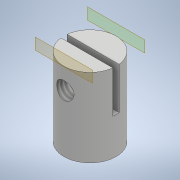
# Autodesk Inventor part: slit-adapter-clear-scope_8_2018
Saved by Autodesk Inventor 2021 (Build 250183000, 183)
## iProperties
Created: 2018-04-16
Part Number: slit-adapter-clear-scope_8_2018
Material: Generic
Document SubType Name: Modeling
Designer: FiolkaLab
Density: 1 g/cm^3
Appearance: Default
Author: FiolkaLab
Autodesk Inventor part; units mm, degrees
ref_plane "YZ Plane" through (0, 0, 0) normal (1, 0, 0) x (0, 1, 0)
ref_plane "XZ Plane" through (0, 0, 0) normal (0, 1, 0) x (-1, 0, 0)
ref_plane "XY Plane" through (0, 0, 0) normal (0, 0, 1) x (1, 0, 0)
sketch "Sketch1" plane through (0, 0, 0) normal (0, 0, 1) x (1, 0, 0)
  circle A0 centre (0, 0) radius 5
  dimension "d0" = 10
  constraints: 1 centre point, 1 coincident
  measures "d0" diameter of A0
extrude "Extrusion1" add sketch "Sketch1" along normal blind 15
sketch "Sketch2" plane through (0, 0, 15) normal (0, 0, 1) x (1, 0, 0)
  line L0 (-4.9749, -0.5) -> (4.9749, -0.5)
  line L1 (4.9749, -0.5) -> (4.9749, 0.5)
  line L2 (4.9749, 0.5) -> (-4.9749, 0.5)
  line L3 (-4.9749, 0.5) -> (-4.9749, -0.5)
  circle A0 centre (0, 0) radius 5 projected
  dimension "d3" = 1
  constraints: 8 end point, 3 point on circle, 2 parallel, 1 horizontal, 1 perpendicular
  measures "d3" distance of L2.end L0.start
sketch "Sketch3" plane through (0, 0, 0) normal (0, 0, -1) x (-1, 0, 0)
  circle A0 centre (0, 0) radius 1.4142
  constraints: 1 centre point, 1 coincident
hole "Hole1" at (0, 0, 0) direction (0, 0, 1) diameter 3.302 depth 7 thread size "8-32 UNC" class "2B" standard "ANSI Unified Screw Threads"
extrude "Extrusion2" add sketch "Sketch2" along normal blind 2 contours L3 L2 L1 L0
ref_plane "Work Plane1" through (-4.9749, 5, 15) normal (0, 1, 0) x (1, 0, 0)
ref_plane "Work Plane2" through (-4.9749, -5, 15) normal (0, -1, 0) x (1, 0, 0)
sketch "Sketch5" plane through (-4.9749, -5, 15) normal (0, -1, 0) x (1, 0, 0)
  circle A0 centre (5, -4) radius 1.0003
  line L0 (9.9499, 0) -> (0, 0) projected
  point P0 (4.9749, -15)
  dimension "d16" = 4
  constraints: 1 centre point
  measures "d16" distance from line of L0 A0.centre
hole "Hole2" at (0.0251, -5, 11) direction (0, 1, 0) diameter 3.302 depth 4.5 thread size "8-32 UNC" class "2B" standard "ANSI Unified Screw Threads"
sketch "Sketch6" plane through (0, 0, 15) normal (0, 0, 1) x (1, 0, 0)
  arc A0 (-4.9749, 0.5) -> (-4.9749, -0.5) centre (0, 0) ccw projected
  line L0 (4.9749, 0.5) -> (4.9749, -0.5) projected
  line L1 (-4.9749, -0.5) -> (4.9749, -0.5)
  line L2 (4.9749, -0.5) -> (4.9749, 0.5)
  line L3 (4.9749, 0.5) -> (-4.9749, 0.5)
  line L4 (-4.9749, 0.5) -> (-4.9749, -0.5)
  constraints: 8 end point, 2 parallel, 1 horizontal, 1 perpendicular
extrude "Extrusion3" add sketch "Sketch6" against normal blind 2 contours L3 L0 L1 L4
sketch "Sketch7" plane through (0, 0, 17) normal (0, 0, 1) x (1, 0, 0)
  line L0 (5, 0.6) -> (-5, 0.6)
  line L1 (-5, 0.6) -> (-5, -0.6)
  line L2 (-5, -0.6) -> (5, -0.6)
  line L3 (5, -0.6) -> (5, 0.6)
  arc A0 (4.9749, -0.5) -> (4.9749, 0.5) centre (0, 0) ccw projected
  arc A1 (-4.9749, 0.5) -> (-4.9749, -0.5) centre (0, 0) ccw projected
  dimension "d35" = 1.2
  dimension "d36" = 0.6
  constraints: 8 end point, 2 parallel, 2 tangent, 1 horizontal, 1 perpendicular
  measures "d35" distance of L0.end L1.end
  measures "d36" distance from line of point (0, 0) L2
extrude "Extrusion4" cut sketch "Sketch7" against normal blind 10
body "Solid1"
